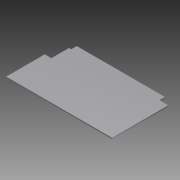
# Autodesk Inventor part: 24in-by-14in_electronics_board
Saved by Autodesk Inventor 2012 (Build 160160000, 160)
## iProperties
Created: 2012-01-09
Part Number: 24in-by-14in_electronics_board
Material: Default
Document SubType Name: Modeling
Designer: William
Density: 1 g/cm^3
Author: William
Autodesk Inventor part; units mm, degrees
ref_plane "YZ Plane" through (0, 0, 0) normal (1, 0, 0) x (0, 1, 0)
ref_plane "XZ Plane" through (0, 0, 0) normal (0, 1, 0) x (-1, 0, 0)
ref_plane "XY Plane" through (0, 0, 0) normal (0, 0, 1) x (1, 0, 0)
sketch "Sketch1" plane through (0, 0, 0) normal (0, 0, 1) x (1, 0, 0)
  line L0 (-379.6568, 188.1861) -> (255.3432, 188.1861)
  line L1 (255.3432, 188.1861) -> (255.3432, 194.5361)
  line L2 (255.3432, 194.5361) -> (-379.6568, 194.5361)
  line L3 (-379.6568, 194.5361) -> (-379.6568, 188.1861)
  point P0 (0, 0)
  dimension "d0" = 635
  dimension "d1" = 6.35
  constraints: 8 end point, 2 parallel, 1 horizontal, 1 perpendicular
  measures "d0" distance of L2.end L1.end
  measures "d1" distance of L1.end L0.end
extrude "Extrusion1" add sketch "Sketch1" along normal blind 355.6
sketch "Sketch2" plane through (-379.6568, 188.1861, 0) normal (0, -1, 0) x (1, 0, 0)
  line L0 (635, 355.6) -> (0, 355.6) projected
  line L1 (0, 0) -> (0, 355.6) projected
  line L2 (0, 0) -> (635, 0) projected
  line L3 (635, 0) -> (635, 355.6) projected
  line L4 (12.7, 355.6) -> (622.3, 355.6)
  line L5 (622.3, 355.6) -> (622.3, 0)
  line L6 (622.3, 0) -> (12.7, 0)
  line L7 (12.7, 0) -> (12.7, 355.6)
  point P0 (379.6568, 0)
  dimension "d4" = 609.6
  dimension "d5" = 355.6
  dimension "d6" = 12.7
  constraints: 8 end point, 2 parallel, 1 horizontal, 1 perpendicular, 1 point on line
  measures "d4" distance of L5.end L6.end
  measures "d5" distance of L6.end L4.start
  measures "d6" distance between parallel lines of L1 L7
extrude "Extrusion2" cut sketch "Sketch2" against normal blind 355.6 contours L3 L2 L5 L0 | L7 L2 L1 L0
sketch "Sketch3" plane through (-366.9568, 194.5361, 0) normal (0, 1, 0) x (1, 0, 0)
  line L0 (0, 0) -> (0, -355.6) projected
  line L1 (609.6, 0) -> (558.8, 0)
  line L2 (558.8, 0) -> (558.8, -31.75)
  line L3 (558.8, -31.75) -> (609.6, -31.75)
  line L4 (609.6, -31.75) -> (609.6, 0)
  line L5 (0, 0) -> (50.8, 0)
  line L6 (50.8, 0) -> (50.8, -31.75)
  line L7 (50.8, -31.75) -> (0, -31.75)
  line L8 (0, -31.75) -> (0, 0)
  line L9 (0, -133.35) -> (38.1, -133.35)
  line L10 (38.1, -133.35) -> (38.1, -31.75)
  line L11 (38.1, -31.75) -> (0, -31.75)
  line L12 (0, -31.75) -> (0, -133.35)
  point P0 (366.9568, 0)
  dimension "d9" = 50.8
  dimension "d10" = 31.75
  dimension "d11" = 50.8
  dimension "d12" = 31.75
  dimension "d13" = 38.1
  dimension "d14" = 101.6
  constraints: 24 end point, 6 parallel, 3 horizontal, 3 perpendicular, 1 point on line
  measures "d9" distance of L3.end L2.end
  measures "d10" distance of L2.end L1.end
  measures "d11" distance of L6.end L7.end
  measures "d12" distance of L5.end L6.end
  measures "d13" distance of L11.end L10.end
  measures "d14" distance of L10.end L9.end
extrude "Extrusion3" cut sketch "Sketch3" against normal blind 25.4
body "Solid1"
